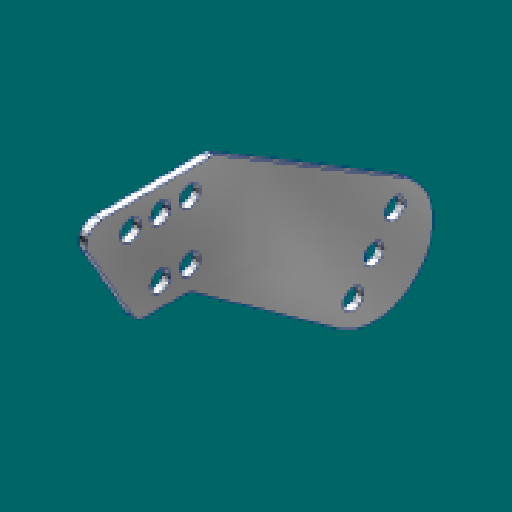
# Autodesk Inventor part: IntakeArm
Saved by Autodesk Inventor 2023.1 (Build 271208000, 208)
## iProperties
Created: 2022-11-06
Part Number: IntakeArm
Material: Aluminum 6061
Document SubType Name: Modeling
Designer: zac-h
Density: 2.7 g/cm^3
Appearance: Aluminum - Flat
Mass: 7.06246 g
Surface Area: 37.7141 cm^2
Volume: 2.61572 cm^3
Author: zac-h
Autodesk Inventor part; units mm, degrees
ref_plane "YZ Plane" through (0, 0, 0) normal (1, 0, 0) x (0, 1, 0)
ref_plane "XZ Plane" through (0, 0, 0) normal (0, 1, 0) x (-1, 0, 0)
ref_plane "XY Plane" through (0, 0, 0) normal (0, 0, 1) x (1, 0, 0)
sketch "Sketch1" plane through (0, 0, 0) normal (1, 0, 0) x (0, 1, 0)
  circle A0 centre (0, 0) radius 2.159
  line L0 (0, 0) -> (0, 39.624) construction
  line L1 (0, 39.624) -> (12.827, 39.624) construction
  line L2 (12.827, 39.624) -> (12.827, 51.054)
  circle A1 centre (0, 0) radius 12.7
  line L3 (12.827, 39.624) -> (-10.3145, 7.4095)
  line L4 (12.827, 51.054) -> (35.687, 51.054) construction
  line L5 (35.687, 51.054) -> (35.687, 34.544)
  line L6 (35.687, 34.544) -> (12.827, 34.544) construction
  line L7 (12.827, 34.544) -> (12.827, 51.054)
  line L8 (35.687, 34.544) -> (10.8726, -6.5633)
  circle A2 centre (30.607, 45.974) radius 2.159
  line L9 (30.607, 45.974) -> (30.607, 33.274) construction
  line L10 (30.607, 45.974) -> (17.907, 45.974) construction
  circle A3 centre (30.607, 39.624) radius 2.159
  circle A4 centre (17.907, 45.974) radius 2.159
  circle A5 centre (17.907, 39.624) radius 2.159
  line L11 (12.827, 51.054) -> (35.687, 64.2522)
  line L12 (35.687, 64.2522) -> (35.687, 51.054)
  circle A6 centre (30.607, 52.324) radius 2.159
  circle A7 centre (6.1887, -4.4457) radius 2.159
  line L13 (0, 0) -> (6.1887, -4.4457) construction
  circle A8 centre (0, 0) radius 7.62 construction
  circle A9 centre (-6.1887, 4.4457) radius 2.159
  dimension "d29" = 15.24
  dimension "d0" = 4.318
  dimension "d1" = 39.624
  dimension "d2" = 11.43
  dimension "d3" = 12.827
  dimension "d5" = 25.4
  dimension "d6" = 22.86
  dimension "d7" = 16.51
  dimension "d8" = 4.318
  dimension "d9" = 5.08
  dimension "d10" = 5.08
  dimension "d11" = 12.7
  dimension "d12" = 12.7
  dimension "d15" = 6.35
  dimension "d18" = 12.7
  dimension "d21" = 30
  dimension "d22" = 6.35
  dimension "d26" = 4.318
  dimension "d32" = 360
  constraints: 28 end point, 9 centre point, 5 vertical, 3 horizontal, 3 perpendicular, 2 coincident, 2 parallel, 2 point on circle, 2 tangent, 1 equal radius, 1 point on line, 1 vertical alignment, 14 other
  measures "d0" diameter of A0
  measures "d1" distance of L0.start L0.end
  measures "d2" distance of L1.end L2.end
  measures "d3" distance of L0.end L1.end
  measures "d5" diameter of A1
  measures "d6" distance of L5.end L6.end
  measures "d7" distance of L4.end L5.end
  measures "d8" diameter of A2
  measures "d9" distance from line of L5 L9.start
  measures "d10" distance from line of L4 L9.start
  measures "d11" distance of L9.start L9.end
  measures "d12" distance of L9.start L10.end
  measures "d15" distance of L9.start A3.centre
  measures "d18" distance of L9.start A4.centre
  measures "d21" angle of L11 L4
  measures "d22" distance of L9.start A6.centre
  measures "d26" diameter of A7
extrude "Extrusion1" add sketch "Sketch1" along normal blind 1.5875
fillet "Fillet1" radius 3.175 4 edges at (0.7937, 12.827, 39.624) (0.7937, 35.687, 34.544) (0.7937, 35.687, 64.2522) (0.7937, 12.827, 51.054)
body "Solid1"
